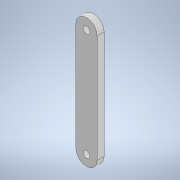
# Autodesk Inventor part: Linkage
Saved by Autodesk Inventor 2022 (Build 260153000, 153)
## iProperties
Created: 2022-04-03
Part Number: Linkage
Material: Generic
Document SubType Name: Modeling
Designer: Nick
Density: 1 g/cm^3
Appearance: Default
Author: Nick
Autodesk Inventor part; units mm, degrees
ref_plane "YZ Plane" through (0, 0, 0) normal (1, 0, 0) x (0, 1, 0)
ref_plane "XZ Plane" through (0, 0, 0) normal (0, 1, 0) x (-1, 0, 0)
ref_plane "XY Plane" through (0, 0, 0) normal (0, 0, 1) x (1, 0, 0)
sketch "Sketch1" plane through (0, 0, 0) normal (0, 0, 1) x (1, 0, 0)
  line L0 (0, 0) -> (9.525, 0)
  line L1 (9.525, 0) -> (9.525, 58.0931)
  line L2 (9.525, 58.0931) -> (0, 58.0931)
  line L3 (0, 58.0931) -> (0, 0)
  circle A0 centre (4.7625, 53.3306) radius 4.7625
  circle A1 centre (4.7625, 4.7625) radius 4.7625
  point P0 (4.7625, 4.7625)
  point P1 (4.7625, 0)
  dimension "d0" = 48.5681
  dimension "d3" = 9.525
  constraints: 8 end point, 6 tangent, 2 centre point, 2 coincident, 2 parallel, 2 vertical alignment, 1 horizontal, 1 midpoint, 1 perpendicular
  measures "d0" distance of point (4.762, 53.331) point (4.762, 4.763)
  measures "d3" distance of L1.end L2.end
extrude "Extrusion1" add sketch "Sketch1" along normal blind 3.175
hole "Hole1" at (4.7625, 4.7625, 0) at (4.7625, 53.3306, 0) direction (0, 0, 1) diameter 3 end through all
fillet "Fillet1" radius 4.7625 4 edges at (9.525, 0, 1.5875) (0, 0, 1.5875) (0, 58.0931, 1.5875) (9.525, 58.0931, 1.5875)
body "Solid1"
